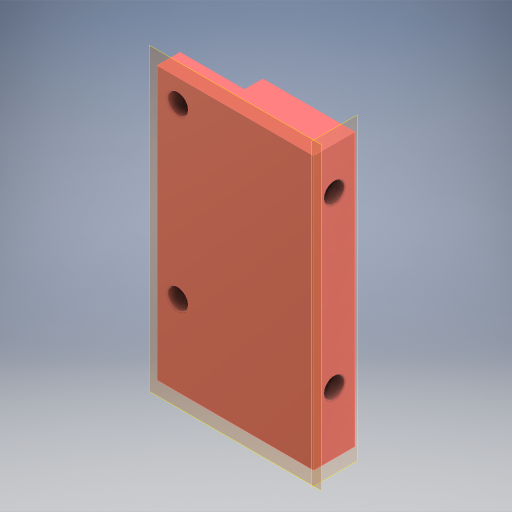
# Autodesk Inventor part: dehind ankle connection_inside
Saved by Autodesk Inventor 2024 (Build 280153000, 153)
## iProperties
Created: 2024-09-16
Part Number: dehind ankle connection_inside
Material: PMMA 플라스틱
Document SubType Name: Modeling
Designer: msi
Density: 1.188 g/cm^3
Appearance: 매끄러움 - 빨간색
Author: msi
Autodesk Inventor part; units mm, degrees
ref_plane "YZ Plane" through (0, 0, 0) normal (1, 0, 0) x (0, 1, 0)
ref_plane "XZ Plane" through (0, 0, 0) normal (0, 1, 0) x (-1, 0, 0)
ref_plane "XY Plane" through (0, 0, 0) normal (0, 0, 1) x (1, 0, 0)
ref_plane "작업 평면1" through (0, 0, 0) normal (0, 0, 1) x (1, 0, 0)
sketch "스케치1" plane through (0, 0, 0) normal (0, 0, 1) x (1, 0, 0)
  line L0 (6.3, 9.65) -> (6.3, 14.85) projected
  line L1 (4.1, 9.65) -> (6.3, 9.65) projected
  line L2 (4.1, 14.85) -> (4.1, 9.65) projected
  line L3 (6.3, 14.85) -> (4.1, 14.85) projected
  line L4 (4.1, -7.15) -> (4.1, -12.35) projected
  line L5 (6.3, -7.15) -> (4.1, -7.15) projected
  line L6 (6.3, -12.35) -> (6.3, -7.15) projected
  line L7 (4.1, -12.35) -> (6.3, -12.35) projected
  line L8 (10.2, -17.75) -> (-10.2, -17.75) projected
  line L9 (10.2, 17.75) -> (10.2, -17.75) projected
  line L10 (-10.2, 17.75) -> (10.2, 17.75) projected
  line L11 (-10.2, -17.75) -> (-10.2, 17.75) projected
  circle A0 centre (-7.5, 14.75) radius 1.35 projected
  circle A1 centre (-7.5, -7.25) radius 1.35 projected
  line L12 (-10.2, 17.75) -> (10.2, 17.75)
  line L13 (10.2, 17.75) -> (10.2, -17.75)
  line L14 (10.2, -17.75) -> (-10.2, -17.75)
  line L15 (-10.2, -17.75) -> (-10.2, 17.75)
  point P0 (0, 0)
  constraints: 8 end point, 2 parallel, 1 horizontal, 1 perpendicular
extrude "돌출1" add sketch "스케치1" against normal blind 3
ref_plane "작업 평면2" through (10.2, 17.75, -3) normal (1, 0, 0) x (0, -1, 0)
sketch "스케치2" plane through (10.2, 17.75, -3) normal (1, 0, 0) x (0, -1, 0)
  circle A0 centre (27.5, -0.3) radius 1.35 projected
  circle A1 centre (5.5, -0.3) radius 1.35 projected
  line L0 (35.5, 2.4) -> (35.5, -3) projected
  line L1 (0, 2.4) -> (35.5, 2.4) projected
  line L2 (0, 2.4) -> (0, -3) projected
  line L3 (0, -3) -> (35.5, -3) projected
  line L4 (0, -3) -> (35.5, -3)
  line L5 (35.5, -3) -> (35.5, 2.4)
  line L6 (35.5, 2.4) -> (0, 2.4)
  line L7 (0, 2.4) -> (0, -3)
  point P0 (17.75, -3)
  constraints: 8 end point, 2 parallel, 1 horizontal, 1 perpendicular
extrude "돌출2" add sketch "스케치2" against normal blind 12
sketch "스케치3" plane through (10.2, -17.75, 0) normal (1, 0, 0) x (0, 0, -1)
  circle A0 centre (2.7, 8) radius 1.35 projected
  circle A1 centre (2.7, 30) radius 1.35 projected
  line L0 (5.4, 0) -> (0, 0) projected
  line L1 (5.4, 35.5) -> (5.4, 0) projected
  line L2 (5.4, 35.5) -> (0, 35.5) projected
  line L3 (0, 35.5) -> (0, 0) projected
  circle A2 centre (2.7, 30) radius 1.35
  circle A3 centre (2.7, 8) radius 1.35
  point P0 (0, 17.75)
  constraints: 2 centre point, 2 coincident, 2 concentric
extrude "돌출3" cut sketch "스케치3" against normal blind 12 contours A0 | A1
